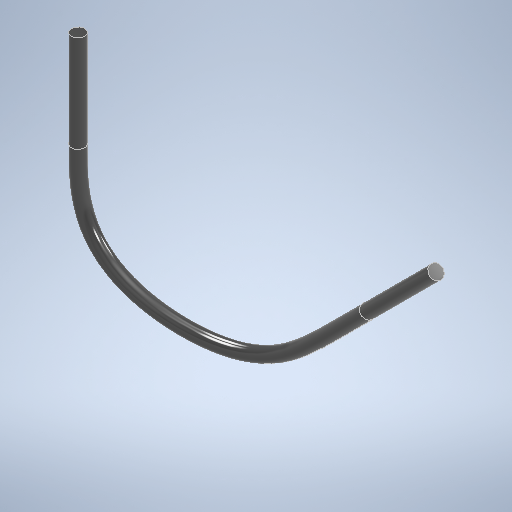
# Autodesk Inventor part: Kabel3
Saved by Autodesk Inventor 2025.2 (Build 292293000, 293)
## iProperties
Created: 2024-11-20
Part Number: Kabel3
Material: Generisch
Document SubType Name: Modeling
Designer: tills
Density: 1 g/cm^3
Appearance: Dunkelgrau
Author: tills
Autodesk Inventor part; units mm, degrees
ref_plane "YZ Plane" through (0, 0, 0) normal (1, 0, 0) x (0, 1, 0)
ref_plane "XZ Plane" through (0, 0, 0) normal (0, 1, 0) x (-1, 0, 0)
ref_plane "XY Plane" through (0, 0, 0) normal (0, 0, 1) x (1, 0, 0)
sketch "Skizze1" plane through (0, 0, 0) normal (0, 0, 1) x (1, 0, 0)
  line L0 (0, 0) -> (0, -50)
  line L1 (150, -50) -> (185.355, -14.645)
  spline S0 degree 4 poles (0, -50) (0, -70.8589) (0, -105.6238) (92.5422, -112.9915) (117.2999, -82.7001) (137.7375, -62.2625) (150, -50) knots 0 0 0 0 0 0.375 0.625 1 1 1 1 1
  point P0 (75, -102.9793)
  dimension "d0" = 50
  dimension "d1" = 45
  dimension "d2" = 150
  dimension "d3" = 35.355
  dimension "d4" = 75
  constraints: 4 end point, 2 vertical, 1 horizontal alignment, 4 other
  measures "d0" distance of L0.start L0.end
  measures "d1" angle of L0 L1
  measures "d2" distance of L0.end L1.start
  measures "d3" horizontal distance of L1.start L1.end
  measures "d4" horizontal distance of L0.end point (75, -102.979)
sketch "Skizze2" plane through (0, 0, 0) normal (0, 1, 0) x (-1, 0, 0)
  circle A0 centre (0, 0) radius 3.5
  dimension "d5" = 7
  constraints: 1 centre point, 1 coincident
  measures "d5" diameter of A0
sweep "Sweeping1" add profiles "Skizze2" path "Skizze1"
